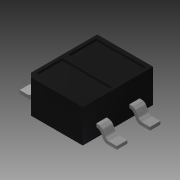
# Autodesk Inventor part: QRE1113
Saved by Autodesk Inventor 2015 SP1 (Build 190203100, 203)
## iProperties
Created: 2015-11-23
Part Number: QRE1113
Material: Типовые
Document SubType Name: Modeling
Designer: danil
Density: 1 g/cm^3
Appearance: Анодированный - черный(1)
Author: danil
Autodesk Inventor part; units mm, degrees
ref_plane "YZ Plane" through (0, 0, 0) normal (1, 0, 0) x (0, 1, 0)
ref_plane "XZ Plane" through (0, 0, 0) normal (0, 1, 0) x (-1, 0, 0)
ref_plane "XY Plane" through (0, 0, 0) normal (0, 0, 1) x (1, 0, 0)
sketch "Эскиз1" plane through (0, 0, 0) normal (0, 0, 1) x (1, 0, 0)
  line L0 (-1.15, -1.7) -> (1.35, -1.7)
  line L1 (1.35, -1.7) -> (1.35, 1.7)
  line L2 (1.35, 1.7) -> (-1.35, 1.7)
  line L3 (-1.35, 1.7) -> (-1.35, -1.5)
  line L4 (-1.35, -1.7) -> (1.35, 1.7) construction
  line L5 (1.35, -1.7) -> (-1.35, 1.7) construction
  line L6 (1.2018, 0.1589) -> (-1.2018, 0.1589)
  line L7 (-1.2018, 0.1589) -> (-1.2018, 1.5134)
  line L8 (-1.2018, 1.5134) -> (1.2018, 1.5134)
  line L9 (1.2018, 1.5134) -> (1.2018, 0.1589)
  line L10 (1.2018, 0.1589) -> (-1.2018, 1.5134) construction
  line L11 (-1.2018, 0.1589) -> (1.2018, 1.5134) construction
  line L12 (-1.15, -1.7) -> (-1.35, -1.5)
  line L13 (1.2018, -1.5318) -> (-1.0018, -1.5318)
  line L14 (-1.2018, -1.3318) -> (-1.2018, -0.1426)
  line L15 (-1.2018, -0.1426) -> (1.2018, -0.1426)
  line L16 (1.2018, -0.1426) -> (1.2018, -1.5318)
  line L17 (1.2018, -1.5318) -> (-1.2018, -0.1426) construction
  line L18 (-1.2018, -1.5318) -> (1.2018, -0.1426) construction
  line L19 (-1.0018, -1.5318) -> (-1.2018, -1.3318)
  point P0 (0, 0)
  point P1 (0, 0.8361)
  point P2 (0, -0.8372)
  dimension "d0" = 2.7
  dimension "d1" = 3.4
  dimension "d2" = 0.2
  dimension "d3" = 0.2
  dimension "d4" = 0.2
  dimension "d5" = 0.2
  constraints: 40 end point, 6 midpoint, 6 parallel, 5 point on line, 3 horizontal, 3 perpendicular, 2 collinear
  measures "d0" distance of L2.end L1.end
  measures "d1" distance of L1.end L0.end
  measures "d2" distance of L0.start L4.start
  measures "d3" distance of L3.end L4.start
  measures "d4" distance of L13.end L18.start
  measures "d5" distance of L14.start L18.start
extrude "Выдавливание1" add sketch "Эскиз1" along normal blind 1.6
extrude "Выдавливание2" add sketch "Эскиз1" along normal blind 1.5 contours L6 L7 L8 L9 | L13 L19 L14 L15 L16
sketch "Эскиз2" plane through (-1.35, 1.7, 0) normal (0, 1, 0) x (1, 0, 0)
  line L0 (0, 0) -> (0, -1.6) projected
  line L1 (0, -0.6) -> (-0.1, -0.6)
  line L2 (-0.3206, -0.4676) -> (-0.4194, -0.2824)
  line L3 (-0.64, -0.15) -> (-1, -0.15)
  line L4 (-1, -0.15) -> (-1, 0)
  line L5 (-1, 0) -> (-0.55, 0)
  line L6 (-0.3294, -0.1324) -> (-0.2306, -0.3176)
  line L7 (-0.01, -0.45) -> (0, -0.45)
  line L8 (0, 0) -> (2.7, 0) projected
  arc A0 (-0.4194, -0.2824) -> (-0.64, -0.15) centre (-0.64, -0.4) ccw
  arc A1 (-0.3206, -0.4676) -> (-0.1, -0.6) centre (-0.1, -0.35) ccw
  arc A2 (-0.2306, -0.3176) -> (-0.01, -0.45) centre (-0.01, -0.2) ccw
  arc A3 (-0.3294, -0.1324) -> (-0.55, 0) centre (-0.55, -0.25) ccw
  line L9 (1.35, 0) -> (1.35, -1.6) construction
  line L10 (2.7, -0.6) -> (2.8, -0.6)
  line L11 (3.0206, -0.4676) -> (3.1194, -0.2824)
  line L12 (3.34, -0.15) -> (3.7, -0.15)
  line L13 (3.7, -0.15) -> (3.7, 0)
  line L14 (3.7, 0) -> (3.25, 0)
  line L15 (3.0294, -0.1324) -> (2.9306, -0.3176)
  line L16 (2.71, -0.45) -> (2.7, -0.45)
  arc A4 (3.34, -0.15) -> (3.1194, -0.2824) centre (3.34, -0.4) ccw
  arc A5 (2.8, -0.6) -> (3.0206, -0.4676) centre (2.8, -0.35) ccw
  arc A6 (2.71, -0.45) -> (2.9306, -0.3176) centre (2.71, -0.2) ccw
  arc A7 (3.25, 0) -> (3.0294, -0.1324) centre (3.25, -0.25) ccw
  line L17 (0, -0.6) -> (0, -0.45)
  line L18 (2.7, -0.6) -> (2.7, -0.45)
  line L19 (2.7, 0) -> (2.7, -1.6) projected
  point P0 (-0.25, -0.6)
  point P1 (-0.4, 0)
  point P2 (2.95, -0.6)
  point P3 (3.1, 0)
  dimension "d10" = 0.25
  dimension "d11" = 0.15
  dimension "d12" = 0.15
  dimension "d13" = 0.15
  dimension "d14" = 0.6
  dimension "d15" = 1
  dimension "d16" = 0.6
  dimension "d17" = 0.25
  constraints: 34 end point, 18 symmetric about line, 16 point on circle, 10 point on line, 8 centre point, 8 tangent, 3 equal radius, 3 parallel, 2 collinear, 2 perpendicular, 2 vertical, 1 horizontal, 4 other
  measures "d10" distance of L1.start point (-0.25, -0.6)
  measures "d11" distance of L3.end L4.end
  measures "d12" distance between parallel lines of L1 L7
  measures "d13" distance between parallel lines of L6 L2
  measures "d14" distance between parallel lines of L8 L1
  measures "d15" distance between parallel lines of L0 L4
  measures "d16" distance of L4.end point (-0.4, 0)
  measures "d17" radius of A0
extrude "Выдавливание3" add sketch "Эскиз2" against normal blind 1.15
extrude "Выдавливание4" cut sketch "Эскиз2" against normal blind 0.65
sketch "Эскиз3" plane through (-1.15, -1.7, 0) normal (0, -1, 0) x (1, 0, 0)
  line L0 (-1.2, 0) -> (-0.75, 0)
  line L1 (3.5, 0) -> (3.05, 0)
  line L2 (-0.2, 0) -> (-0.2, 1.6) projected
  line L3 (2.5, 0) -> (2.5, 1.6) projected
  line L4 (2.5, 0) -> (-0.2, 0) construction
  line L5 (-0.2, 0.6) -> (-0.3, 0.6)
  line L6 (-0.5206, 0.4676) -> (-0.6194, 0.2824)
  line L7 (-0.84, 0.15) -> (-1.2, 0.15)
  line L8 (-1.2, 0.15) -> (-1.2, 0)
  line L9 (-0.5294, 0.1324) -> (-0.4306, 0.3176)
  line L10 (-0.21, 0.45) -> (-0.2, 0.45)
  arc A0 (-0.84, 0.15) -> (-0.6194, 0.2824) centre (-0.84, 0.4) ccw
  arc A1 (-0.3, 0.6) -> (-0.5206, 0.4676) centre (-0.3, 0.35) ccw
  arc A2 (-0.21, 0.45) -> (-0.4306, 0.3176) centre (-0.21, 0.2) ccw
  arc A3 (-0.75, 0) -> (-0.5294, 0.1324) centre (-0.75, 0.25) ccw
  line L11 (1.15, 0) -> (1.15, 0.6) construction
  arc A4 (2.7306, 0.3176) -> (2.51, 0.45) centre (2.51, 0.2) ccw
  arc A5 (2.8206, 0.4676) -> (2.6, 0.6) centre (2.6, 0.35) ccw
  line L12 (2.8294, 0.1324) -> (2.7306, 0.3176)
  line L13 (2.8206, 0.4676) -> (2.9194, 0.2824)
  arc A6 (2.8294, 0.1324) -> (3.05, 0) centre (3.05, 0.25) ccw
  arc A7 (2.9194, 0.2824) -> (3.14, 0.15) centre (3.14, 0.4) ccw
  line L14 (3.14, 0.15) -> (3.5, 0.15)
  line L15 (3.5, 0.15) -> (3.5, 0)
  line L16 (2.5, 0.6) -> (2.6, 0.6)
  line L17 (2.51, 0.45) -> (2.5, 0.45)
  line L18 (-0.2, 0.6) -> (-0.2, 0.45)
  line L19 (2.5, 0.6) -> (2.5, 0.45)
  point P0 (-0.6, 0)
  point P1 (2.9, 0)
  point P2 (-0.45, 0.6)
  point P3 (2.75, 0.6)
  dimension "d28" = 0.6
  constraints: 36 end point, 16 point on circle, 8 centre point, 8 point on line, 1 horizontal, 1 midpoint
  measures "d28" distance of L0.start point (-0.6, 0)
extrude "Выдавливание5" add sketch "Эскиз3" against normal blind 1.15
extrude "Выдавливание6" cut sketch "Эскиз3" against normal blind 0.65
equation "\"d3\" = d2"
equation "\"d5\" = d4"
